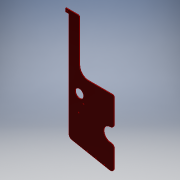
# Autodesk Inventor part: PolyCarb Cover
Saved by Autodesk Inventor 2019.4 (Build 234330000, 330)
## iProperties
Created: 2020-01-29
Part Number: PolyCarb Cover
Material: ABS Plastic
Document SubType Name: Modeling
Designer: admin
Density: 1.06 g/cm^3
Appearance: Red
Mass: 463.116 g
Surface Area: 2263.79 cm^2
Volume: 436.902 cm^3
Author: admin
Autodesk Inventor part; units mm, degrees
ref_plane "YZ Plane" through (0, 0, 0) normal (1, 0, 0) x (0, 1, 0)
ref_plane "XZ Plane" through (0, 0, 0) normal (0, 1, 0) x (-1, 0, 0)
ref_plane "XY Plane" through (0, 0, 0) normal (0, 0, 1) x (1, 0, 0)
sketch "Sketch1" plane through (0, 0, 0) normal (0, 0, 1) x (1, 0, 0)
  line L0 (20, 110) -> (280, 60)
  line L1 (280, 60) -> (280, 208.359)
  arc A0 (280, 277.641) -> (280, 208.359) centre (260, 243) ccw
  line L2 (280, 277.641) -> (280, 450)
  line L3 (280, 450) -> (80, 450)
  line L4 (80, 450) -> (80, 750)
  line L5 (80, 750) -> (0, 750)
  line L6 (0, 750) -> (0, 730)
  line L7 (0, 730) -> (20, 730)
  line L8 (20, 730) -> (20, 110)
  dimension "d3" = 300
  dimension "d4" = 80
  dimension "d6" = 40
  dimension "d7" = 260
  dimension "d8" = 20
  dimension "d9" = 50
  dimension "d11" = 183
  dimension "d21" = 20
  dimension "d32" = 240
  constraints: 18 end point, 3 perpendicular, 3 vertical, 2 point on circle, 1 centre point, 1 collinear, 1 horizontal
  measures "d3" distance of L3.end L4.end
  measures "d4" distance of L4.end L5.end
  measures "d6" radius of A0
  measures "d7" distance between parallel lines of L8 L1
  measures "d8" distance of L6.end L7.end
  measures "d9" vertical distance of L0.start L0.end
  measures "d11" vertical distance of L0.end A0.centre
  measures "d21" distance between parallel lines of L5 L7
  measures "d32" distance from line of L8 A0.centre
extrude "Extrusion1" add sketch "Sketch1" along normal blind 4
fillet "Fillet1" radius 50 1 edges at (80, 450, 2)
fillet "Fillet2" radius 20 2 edges at (280, 208.359, 2) (280, 277.641, 2)
fillet "Fillet3" radius 10 1 edges at (280, 450, 2)
fillet "Fillet4" radius 10 1 edges at (80, 750, 2)
sketch "Sketch2" plane through (0, 0, 4) normal (0, 0, 1) x (1, 0, 0)
  circle A0 centre (10, 740) radius 2.75
  line L0 (0, 750) -> (0, 730) projected
  line L1 (70, 750) -> (0, 750) projected
  point P0 (0, 0)
  dimension "d16" = 5.5
  dimension "d17" = 10
  dimension "d18" = 10
  constraints: 1 centre point
  measures "d16" diameter of A0
  measures "d17" distance from line of L0 A0.centre
  measures "d18" distance from line of L1 A0.centre
extrude "Extrusion2" cut sketch "Sketch2" against normal through all
fillet "Fillet5" radius 2 2 edges at (0, 730, 2) (0, 750, 2)
sketch "Sketch3" plane through (0, 0, 4) normal (0, 0, 1) x (1, 0, 0)
  line L0 (126.7994, 95.5716) -> (225, 76.6869) construction
  line L1 (20, 110) -> (280, 60) projected
  circle A0 centre (126.7994, 95.5716) radius 2.75
  circle A1 centre (225, 76.6869) radius 2.75
  circle A2 centre (175.8997, 86.1292) radius 2.75
  line L2 (280, 60) -> (280, 183) projected
  point P0 (0, 0)
  dimension "d23" = 6
  dimension "d24" = 5.5
  dimension "d25" = 5.5
  dimension "d26" = 5.5
  dimension "d27" = 100
  dimension "d28" = 55
  constraints: 3 centre point, 2 coincident, 2 end point, 1 midpoint, 1 parallel
  measures "d23" distance between parallel lines of L1 L0
  measures "d24" diameter of A0
  measures "d25" diameter of A1
  measures "d26" diameter of A2
  measures "d27" distance of L0.start L0.end
  measures "d28" distance from line of L2 A1.centre
extrude "Extrusion3" cut sketch "Sketch3" against normal through all
fillet "Fillet6" radius 20 2 edges at (280, 60, 2) (20, 110, 2)
sketch "Sketch4" plane through (0, 0, 0) normal (0, 0, -1) x (-1, 0, 0)
  circle A0 centre (-80, 360) radius 25
  line L0 (-270, 450) -> (-130, 450) projected
  line L1 (-280, 303) -> (-280, 440) projected
  point P0 (0, 0)
  dimension "d33" = 50
  dimension "d34" = 90
  dimension "d35" = 200
  constraints: 1 centre point
  measures "d33" diameter of A0
  measures "d34" distance from line of L0 A0.centre
  measures "d35" distance from line of L1 A0.centre
extrude "Extrusion4" cut sketch "Sketch4" against normal through all
sketch "Sketch5" plane through (0, 0, 0) normal (0, 0, -1) x (-1, 0, 0)
  circle A0 centre (-104.34, 320.506) radius 3.429
  circle A1 centre (-76.4, 263.356) radius 3.429
  point P0 (0, 0)
  constraints: 2 centre point, 4 other
extrude "Extrusion5" cut sketch "Sketch5" against normal through all
equation "\"d36\" = d34"
body "Solid1"
